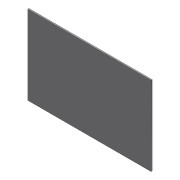
# Autodesk Inventor part: ElectronicsBoardConcept
Saved by Autodesk Inventor 2012 (Build 160160000, 160)
## iProperties
Created: 2012-01-17
Part Number: ElectronicsBoardConcept
Material: Default
Document SubType Name: Modeling
Designer: JesseK
Density: 1 g/cm^3
Author: JesseK
Autodesk Inventor part; units mm, degrees
ref_plane "YZ Plane" through (0, 0, 0) normal (1, 0, 0) x (0, 1, 0)
ref_plane "XZ Plane" through (0, 0, 0) normal (0, 1, 0) x (-1, 0, 0)
ref_plane "XY Plane" through (0, 0, 0) normal (0, 0, 1) x (1, 0, 0)
sketch "Sketch1" plane through (0, 0, 0) normal (0, 0, 1) x (1, 0, 0)
  line L0 (-163.1958, -21.6989) -> (-163.1958, 384.7011)
  line L1 (-163.1958, 384.7011) -> (471.8042, 384.7011)
  line L2 (471.8042, 384.7011) -> (471.8042, -21.6989)
  line L3 (471.8042, -21.6989) -> (-163.1958, -21.6989)
  point P0 (0, 0)
  dimension "d0" = 635
  dimension "d1" = 635
  dimension "d2" = 406.4
  constraints: 8 end point, 2 horizontal, 1 parallel
  measures "d0" distance of L0.end L1.end
  measures "d1" distance of L2.end L0.start
  measures "d2" distance between parallel lines of L3 L1
extrude "Extrusion1" add sketch "Sketch1" along normal blind 6.35
body "Solid1"
